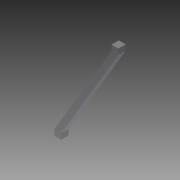
# Autodesk Inventor part: 1Piecelongsupport_v1
Saved by Autodesk Inventor 2013 (Build 170138000, 138)
## iProperties
Created: 2013-01-19
Part Number: 1Piecelongsupport_v1
Material: Polycarbonate, Clear
Document SubType Name: Modeling
Designer: motoennies
Density: 1.2 g/cm^3
Mass: 17.2556 g
Surface Area: 64.846 cm^2
Volume: 14.3796 cm^3
Author: motoennies
Autodesk Inventor part; units mm, degrees
ref_plane "YZ Plane" through (0, 0, 0) normal (1, 0, 0) x (0, 1, 0)
ref_plane "XZ Plane" through (0, 0, 0) normal (0, 1, 0) x (-1, 0, 0)
ref_plane "XY Plane" through (0, 0, 0) normal (0, 0, 1) x (1, 0, 0)
sketch "Sketch1" plane through (0, 0, 0) normal (0, 0, 1) x (1, 0, 0)
  line L0 (0, 0) -> (9.525, 0)
  line L1 (9.525, 0) -> (9.525, 7.62)
  line L2 (0, 0) -> (0, 7.62)
  line L3 (79.121, 140.97) -> (79.121, 148.59)
  line L4 (79.121, 148.59) -> (88.646, 148.59)
  line L5 (88.646, 148.59) -> (88.646, 140.97)
  line L6 (79.121, 140.97) -> (0, 7.62)
  line L7 (9.525, 7.62) -> (88.646, 140.97)
  dimension "d0" = 9.525
  dimension "d1" = 7.62
  dimension "d2" = 7.62
  dimension "d3" = 9.525
  dimension "d4" = 69.596
  dimension "d5" = 133.35
  dimension "d6" = 7.62
  constraints: 16 end point, 3 parallel, 3 perpendicular, 1 horizontal
  measures "d0" distance of L0.start L0.end
  measures "d1" distance of L0.end L1.end
  measures "d2" distance of L3.start L3.end
  measures "d3" distance of L3.end L4.end
  measures "d4" distance between parallel lines of L1 L3
  measures "d5" vertical distance of L3.start L2.end
  measures "d6" distance from line of L5.end L4
extrude "Extrusion1" add sketch "Sketch1" along normal blind 10.16
body "Solid1"
